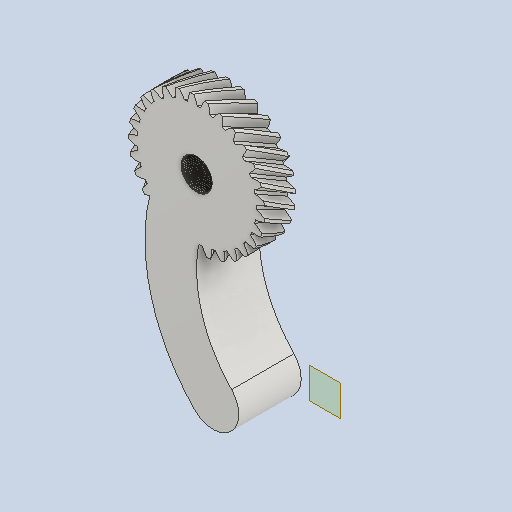
# Autodesk Inventor part: Spur Gear2
Saved by Autodesk Inventor 2024 (Build 280153000, 153)
## iProperties
CustomPartVersion: 1
Created: 2023-09-14
Part Number: Spur Gear2
Material: Steel
Document SubType Name: Modeling
Designer: jebes windows
Categories: <?xml version="1.0" encoding="UTF-16"?> <MemberInstance><Categories><FamilyTemplate><FamilyTemplateParameter ValueType="xs:double" Id="1" ObjectReferenceKey="da_z" ObjectType="kUserParameterObject"/><FamilyTemplateParameter ValueType="xs:double" Id="2" ObjectReferenceKey="da_b" ObjectType="kUserParameterObject"/><FamilyTemplateParameter ValueType="xs:double" Id="3" ObjectReferenceKey="da_beta" ObjectType="kUserParameterObject"/><FamilyTemplateParameter ValueType="xs:double" Id="4" ObjectReferenceKey="da_da" ObjectType="kUserParameterObject"/><FamilyTemplateParameter ValueType="xs:double" Id="5" ObjectReferenceKey="da_aw" ObjectType="kUserParameterObject"/><FamilyTemplateParameter ValueType="xs:string" Id="6" ObjectReferenceKey="EAIAABAAAACIAQAAAAAAAIAAAAAAAAAA" ObjectType="83910656" SubObjectId="SurfaceGeometry"/></FamilyTemplate><ParamToTemplateMap><ParamToTemplate CategoryParameter="//CategoryParameter[@InternalName='046C89C9-8512-4d59-83FE-43B91F4F132A']" TemplateParameter="1"/><ParamToTemplate CategoryParameter="//CategoryParameter[@InternalName='2552DF32-E462-4b46-AEBF-C6C7768E72AC']" TemplateParameter="2"/><ParamToTemplate CategoryParameter="//CategoryParameter[@InternalName='C9EE641D-15FC-4fae-A226-E94C4372FDD7']" TemplateParameter="3"/><ParamToTemplate><ParamToTemplate CategoryParameter="//CategoryParameter[@InternalName='00B6519A-459B-49c7-AD84-2E56D39A5744']" ConstantValue="0.433554"/></ParamToTemplate><ParamToTemplate><ParamToTemplate CategoryParameter="//CategoryParameter[@InternalName='04B31F0E-C7A6-4894-AA32-9629BEFACF47']" ConstantValue="1.000000"/></ParamToTemplate><ParamToTemplate><ParamToTemplate CategoryParameter="//CategoryParameter[@InternalName='43CBEC2E-7847-49e7-A936-2F7889FCB2D9']" ConstantValue="0.250000"/></ParamToTemplate><ParamToTemplate><ParamToTemplate CategoryParameter="//CategoryParameter[@InternalName='B1EFC894-105D-4ebd-86BF-FA20ED196853']" ConstantValue="0.302500"/></ParamToTemplate><ParamToTemplate><ParamToTemplate CategoryParameter="//CategoryParameter[@InternalName='51175063-3D10-4879-93E8-6246FE8B403D']" ConstantValue="2060000000.000000"/></ParamToTemplate><ParamToTemplate><ParamToTemplate CategoryParameter="//CategoryParameter[@InternalName='A3A52E27-4454-46a9-B0BD-C932399B70AF']" ConstantValue="0.300000"/></ParamToTemplate><ParamToTemplate><ParamToTemplate CategoryParameter="//CategoryParameter[@InternalName='91B76062-C214-41d9-B1B9-14D2AB99603D']" ConstantValue="0.060000"/></ParamToTemplate><ParamToTemplate><ParamToTemplate CategoryParameter="//CategoryParameter[@InternalName='374E806E-8B8A-4dda-A9AA-1039D6500AD2']" ConstantValue="16.666667"/></ParamToTemplate><ParamToTemplate><ParamToTemplate CategoryParameter="//CategoryParameter[@InternalName='2D373A89-B862-43d6-8D0B-0CBF12AB9F6C']" ConstantValue="0.436332"/></ParamToTemplate><ParamToTemplate CategoryParameter="//CategoryParameter[@InternalName='37777632-D6A2-4fac-9D53-DB8ACD95C989']" TemplateParameter="4"/><ParamToTemplate CategoryParameter="//CategoryParameter[@InternalName='FD1017F1-B727-4f7e-9707-0F86F1FF9423']" TemplateParameter="5"/><ParamToTemplate><ParamToTemplate CategoryParameter="//CategoryParameter[@InternalName='9E1B4470-B2D3-4ff1-B813-535BB4CDF51A']" ConstantValue="3520000.000000"/></ParamToTemplate><ParamToTemplate><ParamToTemplate CategoryParameter="//CategoryParameter[@InternalName='F8452263-BFF6-458c-9FB1-07C4B99E95CD']" ConstantValue="11400000.000000"/></ParamToTemplate><ParamToTemplate><ParamToTemplate CategoryParameter="//CategoryParameter[@InternalName='3E3BB259-FD49-497f-8171-6EBC954A3479']" ConstantValue="2.000000"/></ParamToTemplate><ParamToTemplate CategoryParameter="//CategoryParameter[@InternalName='27C3BAF2-7550-4e4b-AE2C-0DB134B7D9B7']" TemplateParameter="6"/></ParamToTemplateMap><Category DisplayName="Gear" InternalName="DC85795E-93AB-48d5-8EEE-5A27447B64BD" Mnemonic="Gear"><CategoryParameter DisplayName="z" InternalName="046C89C9-8512-4d59-83FE-43B91F4F132A" Mnemonic="z"/><CategoryParameter DisplayName="b" InternalName="2552DF32-E462-4b46-AEBF-C6C7768E72AC" Mnemonic="b"/><CategoryParameter DisplayName="||b|" InternalName="C9EE641D-15FC-4fae-A226-E94C4372FDD7" Mnemonic="beta"/><CategoryParameter DisplayName="x" InternalName="00B6519A-459B-49c7-AD84-2E56D39A5744" Mnemonic="x"/><CategoryParameter DisplayName="a*" InternalName="04B31F0E-C7A6-4894-AA32-9629BEFACF47" Mnemonic="a"/><CategoryParameter DisplayName="c*" InternalName="43CBEC2E-7847-49e7-A936-2F7889FCB2D9" Mnemonic="c"/><CategoryParameter DisplayName="r|.f|*" InternalName="B1EFC894-105D-4ebd-86BF-FA20ED196853" Mnemonic="rf"/><CategoryParameter DisplayName="E" InternalName="51175063-3D10-4879-93E8-6246FE8B403D" Mnemonic="E"/><CategoryParameter DisplayName="||m|" InternalName="A3A52E27-4454-46a9-B0BD-C932399B70AF" Mnemonic="mi"/><Category DisplayName="SpurGear" InternalName="26C5A22E-A91E-4dfd-A3B3-23CCAFAE1764" Mnemonic="SpurGear"><CategoryParameter DisplayName="m" InternalName="91B76062-C214-41d9-B1B9-14D2AB99603D" Mnemonic="m"/><CategoryParameter DisplayName="P" InternalName="374E806E-8B8A-4dda-A9AA-1039D6500AD2" Mnemonic="PP"/><CategoryParameter DisplayName="||a|" InternalName="2D373A89-B862-43d6-8D0B-0CBF12AB9F6C" Mnemonic="alpha"/><CategoryParameter DisplayName="d|.a|" InternalName="37777632-D6A2-4fac-9D53-DB8ACD95C989" Mnemonic="da"/><CategoryParameter DisplayName="a|.w|" InternalName="FD1017F1-B727-4f7e-9707-0F86F1FF9423" Mnemonic="aw"/><CategoryParameter DisplayName="||s||.Flim|" InternalName="9E1B4470-B2D3-4ff1-B813-535BB4CDF51A" Mnemonic="sFlim"/><CategoryParameter DisplayName="||s||.Hlim|" InternalName="F8452263-BFF6-458c-9FB1-07C4B99E95CD" Mnemonic="sHlim"/><CategoryParameter DisplayName="type" InternalName="3E3BB259-FD49-497f-8171-6EBC954A3479" Mnemonic="type"/><CategoryParameter DisplayName="PitchDiameter" InternalName="27C3BAF2-7550-4e4b-AE2C-0DB134B7D9B7" Mnemonic="IDS_PITCHDIAM"/></Category></Category></Categories></MemberInstance>
Density: 1 g/cm^3
Appearance: Steel
Author: jebes windows
## iProperties of the stored document Spur Gear22_3DPrint.ipt
Created: 2023-09-14
Part Number: Spur Gear22_3DPrint
Material: Generic
Document SubType Name: Modeling
Designer: jebes windows
Density: 1 g/cm^3
Appearance: Default
Author: jebes windows
Autodesk Inventor part; units mm, degrees
ref_plane "YZ Plane" through (0, 0, 0) normal (1, 0, 0) x (0, 1, 0)
ref_plane "XZ Plane" through (0, 0, 0) normal (0, 1, 0) x (-1, 0, 0)
ref_plane "XY Plane" through (0, 0, 0) normal (0, 0, 1) x (1, 0, 0)
sketch "Sketch1" plane through (0, 0, 0) normal (0, 0, 1) x (1, 0, 0)
  circle A0 centre (0, 0) radius 10.9005
  dimension "d0" = 21.801
  constraints: 1 centre point
  measures "d0" diameter of A0
extrude "Extrusion1" add sketch "Sketch1" along normal blind 5
ref_plane "Work Plane2" through (0, 0, 2.5) normal (0, 0, 1) x (1, 0, 0)
sketch "Sketch2" plane through (0, 0, 0) normal (0, 0, -1) x (-1, 0, 0)
  circle A0 centre (0, 0) radius 10.9005 projected
  circle A1 centre (0, 0) radius 10.0459
  dimension "d3" = 20.0918
  constraints: 1 centre point, 1 coincident
  measures "d3" diameter of A1
surface extrude "Pitch Diameter" sketch "Sketch2" against normal through all shown no curves A1
ref_plane "Work Plane8" through (0, 0, 0) normal (0.994138, 0.108119, 0) x (0, 0, 1)
ref_plane "Work Plane9" through (0, 0, 0) normal (1, 0, 0) x (0, 1, 0)
spur gear teeth "Spur Gear" teeth 29 pitch diameter 20.0918 tip diameter 21.801 root diameter 19.1121 face width 5 helix angle 30 hand right start plane through (0, 0, 0) normal (0, 0, -1) x (-1, 0, 0)
sketch "Sketch3" plane through (0, 0, 0) normal (0, 0, -1) x (-1, 0, 0)
  circle A0 centre (0, 0) radius 2.5
  dimension "d49" = 5
  constraints: 1 centre point, 1 coincident
  measures "d49" diameter of A0
extrude "Extrusion2" cut sketch "Sketch3" against normal blind 10
ref_plane "Work Plane11" through (17.5512, -23.0514, 1.9) normal (0, 0, -1) x (0, 1, 0)
sketch "Sketch4" plane through (17.5512, -23.0514, 1.9) normal (0, 0, -1) x (0, 1, 0)
  line L0 (25.1983, -18.5069) -> (25.3277, -18.4572) projected
  arc A0 (25.3277, -18.4572) -> (25.3493, -18.4008) centre (23.0514, -17.5512) ccw projected
  line L1 (25.3493, -18.4008) -> (25.2864, -18.2773) projected
  line L2 (25.2864, -18.2773) -> (25.4099, -18.2143) projected
  arc A1 (25.4099, -18.2143) -> (25.4256, -18.1559) centre (23.0514, -17.5512) ccw projected
  line L3 (25.4256, -18.1559) -> (25.35, -18.0397) projected
  line L4 (25.35, -18.0397) -> (25.4663, -17.9641) projected
  arc A2 (25.4663, -17.9641) -> (25.4758, -17.9045) centre (23.0514, -17.5512) ccw projected
  line L5 (25.4758, -17.9045) -> (25.3885, -17.7967) projected
  line L6 (25.3885, -17.7967) -> (25.4963, -17.7095) projected
  arc A3 (25.4963, -17.7095) -> (25.4994, -17.6491) centre (23.0514, -17.5512) ccw projected
  line L7 (25.4994, -17.6491) -> (25.4014, -17.5511) projected
  line L8 (25.4014, -17.5511) -> (25.4994, -17.453) projected
  arc A4 (25.4994, -17.453) -> (25.4962, -17.3927) centre (23.0514, -17.5512) ccw projected
  line L9 (25.4962, -17.3927) -> (25.3885, -17.3054) projected
  line L10 (25.3885, -17.3054) -> (25.4757, -17.1977) projected
  arc A5 (25.4757, -17.1977) -> (25.4663, -17.138) centre (23.0514, -17.5512) ccw projected
  line L11 (25.4663, -17.138) -> (25.35, -17.0625) projected
  line L12 (25.35, -17.0625) -> (25.4255, -16.9462) projected
  arc A6 (25.4255, -16.9462) -> (25.4099, -16.8878) centre (23.0514, -17.5512) ccw projected
  line L13 (25.4099, -16.8878) -> (25.2863, -16.8249) projected
  line L14 (25.2863, -16.8249) -> (25.3493, -16.7014) projected
  arc A7 (25.3493, -16.7014) -> (25.3276, -16.6449) centre (23.0514, -17.5512) ccw projected
  line L15 (25.3276, -16.6449) -> (25.1982, -16.5953) projected
  line L16 (25.1982, -16.5953) -> (25.2478, -16.4658) projected
  arc A8 (25.2478, -16.4658) -> (25.2204, -16.412) centre (23.0514, -17.5512) ccw projected
  line L17 (25.2204, -16.412) -> (25.0865, -16.3761) projected
  line L18 (25.0865, -16.3761) -> (25.1224, -16.2422) projected
  circle A9 centre (23.0514, -17.5512) radius 2.5 projected
  circle A10 centre (23.0514, -17.5512) radius 0.8 projected
  arc A11 (25.1224, -16.2422) -> (25.0894, -16.1915) centre (23.0514, -17.5512) ccw projected
  line L19 (25.0894, -16.1915) -> (24.9525, -16.1698) projected
  line L20 (24.9525, -16.1698) -> (24.9742, -16.0329) projected
  arc A12 (24.9742, -16.0329) -> (24.9361, -15.9859) centre (23.0514, -17.5512) ccw projected
  line L21 (24.9361, -15.9859) -> (24.7977, -15.9786) projected
  line L22 (24.7977, -15.9786) -> (24.8049, -15.8402) projected
  arc A13 (24.8049, -15.8402) -> (24.7622, -15.7975) centre (23.0514, -17.5512) ccw projected
  circle A14 centre (23.0514, -17.5512) radius 2.5 projected
  circle A15 centre (23.0514, -17.5512) radius 0.8 projected
  line L23 (24.7622, -15.7975) -> (24.6237, -15.8047) projected
  line L24 (24.6237, -15.8047) -> (24.6165, -15.6663) projected
  arc A16 (24.6165, -15.6663) -> (24.5695, -15.6282) centre (23.0514, -17.5512) ccw projected
  line L25 (24.5695, -15.6282) -> (24.4326, -15.6499) projected
  line L26 (24.4326, -15.6499) -> (24.4109, -15.513) projected
  arc A17 (24.4109, -15.513) -> (24.3602, -15.4801) centre (23.0514, -17.5512) ccw projected
  line L27 (24.3602, -15.4801) -> (24.2263, -15.516) projected
  line L28 (24.2263, -15.516) -> (24.1904, -15.382) projected
  arc A18 (24.1904, -15.382) -> (24.1365, -15.3546) centre (23.0514, -17.5512) ccw projected
  line L29 (24.1365, -15.3546) -> (24.0071, -15.4043) projected
  line L30 (24.0071, -15.4043) -> (23.9574, -15.2749) projected
  arc A19 (23.9574, -15.2749) -> (23.901, -15.2532) centre (23.0514, -17.5512) ccw projected
  line L31 (23.901, -15.2532) -> (23.7775, -15.3162) projected
  line L32 (23.7775, -15.3162) -> (23.7145, -15.1926) projected
  arc A20 (23.7145, -15.1926) -> (23.6561, -15.177) centre (23.0514, -17.5512) ccw projected
  line L33 (23.6561, -15.177) -> (23.5399, -15.2525) projected
  line L34 (23.5399, -15.2525) -> (23.4643, -15.1362) projected
  arc A21 (23.4643, -15.1362) -> (23.4046, -15.1268) centre (23.0514, -17.5512) ccw projected
  line L35 (23.4046, -15.1268) -> (23.2969, -15.214) projected
  circle A22 centre (23.0514, -17.5512) radius 2.5 projected
  circle A23 centre (23.0514, -17.5512) radius 0.8 projected
  line L36 (23.2969, -15.214) -> (23.2096, -15.1063) projected
  arc A24 (23.2096, -15.1063) -> (23.1493, -15.1031) centre (23.0514, -17.5512) ccw projected
  line L37 (23.1493, -15.1031) -> (23.0513, -15.2012) projected
  line L38 (23.0513, -15.2012) -> (22.9532, -15.1032) projected
  arc A25 (22.9532, -15.1032) -> (22.8929, -15.1063) centre (23.0514, -17.5512) ccw projected
  line L39 (22.8929, -15.1063) -> (22.8056, -15.2141) projected
  line L40 (22.8056, -15.2141) -> (22.6979, -15.1268) projected
  arc A26 (22.6979, -15.1268) -> (22.6382, -15.1363) centre (23.0514, -17.5512) ccw projected
  line L41 (22.6382, -15.1363) -> (22.5627, -15.2526) projected
  line L42 (22.5627, -15.2526) -> (22.4464, -15.1771) projected
  arc A27 (22.4464, -15.1771) -> (22.388, -15.1927) centre (23.0514, -17.5512) ccw projected
  line L43 (22.388, -15.1927) -> (22.3251, -15.3162) projected
  line L44 (22.3251, -15.3162) -> (22.2015, -15.2533) projected
  arc A28 (22.2015, -15.2533) -> (22.1451, -15.275) centre (23.0514, -17.5512) ccw projected
  line L45 (22.1451, -15.275) -> (22.0954, -15.4044) projected
  circle A29 centre (23.0514, -17.5512) radius 2.5 projected
  circle A30 centre (23.0514, -17.5512) radius 0.8 projected
  line L46 (22.0954, -15.4044) -> (21.966, -15.3547) projected
  arc A31 (21.966, -15.3547) -> (21.9122, -15.3822) centre (23.0514, -17.5512) ccw projected
  line L47 (21.9122, -15.3822) -> (21.8763, -15.5161) projected
  line L48 (21.8763, -15.5161) -> (21.7424, -15.4802) projected
  arc A32 (21.7424, -15.4802) -> (21.6917, -15.5131) centre (23.0514, -17.5512) ccw projected
  line L49 (21.6917, -15.5131) -> (21.67, -15.6501) projected
  line L50 (21.67, -15.6501) -> (21.533, -15.6284) projected
  arc A33 (21.533, -15.6284) -> (21.4861, -15.6664) centre (23.0514, -17.5512) ccw projected
  line L51 (21.4861, -15.6664) -> (21.4788, -15.8049) projected
  line L52 (21.4788, -15.8049) -> (21.3404, -15.7976) projected
  arc A34 (21.3404, -15.7976) -> (21.2976, -15.8404) centre (23.0514, -17.5512) ccw projected
  line L53 (21.2976, -15.8404) -> (21.3049, -15.9788) projected
  line L54 (21.3049, -15.9788) -> (21.1665, -15.9861) projected
  arc A35 (21.1665, -15.9861) -> (21.1284, -16.033) centre (23.0514, -17.5512) ccw projected
  line L55 (21.1284, -16.033) -> (21.1501, -16.17) projected
  line L56 (21.1501, -16.17) -> (21.0132, -16.1917) projected
  arc A36 (21.0132, -16.1917) -> (20.9803, -16.2424) centre (23.0514, -17.5512) ccw projected
  line L57 (20.9803, -16.2424) -> (21.0162, -16.3763) projected
  line L58 (21.0162, -16.3763) -> (20.8822, -16.4122) projected
  circle A37 centre (23.0514, -17.5512) radius 2.5 projected
  circle A38 centre (23.0514, -17.5512) radius 0.8 projected
  arc A39 (20.8822, -16.4122) -> (20.8548, -16.466) centre (23.0514, -17.5512) ccw projected
  line L59 (20.8548, -16.466) -> (20.9045, -16.5955) projected
  line L60 (20.9045, -16.5955) -> (20.7751, -16.6452) projected
  arc A40 (20.7751, -16.6452) -> (20.7534, -16.7016) centre (23.0514, -17.5512) ccw projected
  line L61 (20.7534, -16.7016) -> (20.8164, -16.8251) projected
  line L62 (20.8164, -16.8251) -> (20.6928, -16.8881) projected
  circle A41 centre (23.0514, -17.5512) radius 2.5 projected
  circle A42 centre (23.0514, -17.5512) radius 0.8 projected
  arc A43 (20.6928, -16.8881) -> (20.6772, -16.9464) centre (23.0514, -17.5512) ccw projected
  line L63 (20.6772, -16.9464) -> (20.7527, -17.0627) projected
  line L64 (20.7527, -17.0627) -> (20.6364, -17.1382) projected
  arc A44 (20.6364, -17.1382) -> (20.627, -17.1979) centre (23.0514, -17.5512) ccw projected
  line L65 (20.627, -17.1979) -> (20.7142, -17.3057) projected
  line L66 (20.7142, -17.3057) -> (20.6065, -17.3929) projected
  arc A45 (20.6065, -17.3929) -> (20.6033, -17.4533) centre (23.0514, -17.5512) ccw projected
  line L67 (20.6033, -17.4533) -> (20.7014, -17.5513) projected
  line L68 (20.7014, -17.5513) -> (20.6033, -17.6493) projected
  arc A46 (20.6033, -17.6493) -> (20.6065, -17.7097) centre (23.0514, -17.5512) ccw projected
  line L69 (20.6065, -17.7097) -> (20.7143, -17.7969) projected
  line L70 (20.7143, -17.7969) -> (20.627, -17.9047) projected
  arc A47 (20.627, -17.9047) -> (20.6365, -17.9644) centre (23.0514, -17.5512) ccw projected
  line L71 (20.6365, -17.9644) -> (20.7528, -18.0399) projected
  line L72 (20.7528, -18.0399) -> (20.6772, -18.1562) projected
  arc A48 (20.6772, -18.1562) -> (20.6929, -18.2145) centre (23.0514, -17.5512) ccw projected
  line L73 (20.6929, -18.2145) -> (20.8164, -18.2775) projected
  line L74 (20.8164, -18.2775) -> (20.7535, -18.401) projected
  arc A49 (20.7535, -18.401) -> (20.7752, -18.4574) centre (23.0514, -17.5512) ccw projected
  line L75 (20.7752, -18.4574) -> (20.9046, -18.5071) projected
  line L76 (20.9046, -18.5071) -> (20.8549, -18.6366) projected
  arc A50 (20.8549, -18.6366) -> (20.8823, -18.6904) centre (23.0514, -17.5512) ccw projected
  line L77 (20.8823, -18.6904) -> (21.0163, -18.7263) projected
  line L78 (21.0163, -18.7263) -> (20.9804, -18.8602) projected
  arc A51 (20.9804, -18.8602) -> (21.0133, -18.9109) centre (23.0514, -17.5512) ccw projected
  line L79 (21.0133, -18.9109) -> (21.1503, -18.9326) projected
  line L80 (21.1503, -18.9326) -> (21.1286, -19.0695) projected
  arc A52 (21.1286, -19.0695) -> (21.1666, -19.1165) centre (23.0514, -17.5512) ccw projected
  line L81 (21.1666, -19.1165) -> (21.3051, -19.1237) projected
  line L82 (21.3051, -19.1237) -> (21.2978, -19.2622) projected
  arc A53 (21.2978, -19.2622) -> (21.3405, -19.3049) centre (23.0514, -17.5512) ccw projected
  line L83 (21.3405, -19.3049) -> (21.479, -19.2977) projected
  line L84 (21.479, -19.2977) -> (21.4863, -19.4361) projected
  arc A54 (21.4863, -19.4361) -> (21.5332, -19.4741) centre (23.0514, -17.5512) ccw projected
  line L85 (21.5332, -19.4741) -> (21.6702, -19.4524) projected
  line L86 (21.6702, -19.4524) -> (21.6919, -19.5894) projected
  arc A55 (21.6919, -19.5894) -> (21.7426, -19.6223) centre (23.0514, -17.5512) ccw projected
  line L87 (21.7426, -19.6223) -> (21.8765, -19.5864) projected
  line L88 (21.8765, -19.5864) -> (21.9124, -19.7203) projected
  arc A56 (21.9124, -19.7203) -> (21.9662, -19.7478) centre (23.0514, -17.5512) ccw projected
  line L89 (21.9662, -19.7478) -> (22.0956, -19.6981) projected
  line L90 (22.0956, -19.6981) -> (22.1453, -19.8275) projected
  arc A57 (22.1453, -19.8275) -> (22.2018, -19.8492) centre (23.0514, -17.5512) ccw projected
  line L91 (22.2018, -19.8492) -> (22.3253, -19.7862) projected
  line L92 (22.3253, -19.7862) -> (22.3882, -19.9097) projected
  arc A58 (22.3882, -19.9097) -> (22.4466, -19.9254) centre (23.0514, -17.5512) ccw projected
  line L93 (22.4466, -19.9254) -> (22.5629, -19.8499) projected
  line L94 (22.5629, -19.8499) -> (22.6384, -19.9661) projected
  arc A59 (22.6384, -19.9661) -> (22.6981, -19.9756) centre (23.0514, -17.5512) ccw projected
  line L95 (22.6981, -19.9756) -> (22.8058, -19.8883) projected
  line L96 (22.8058, -19.8883) -> (22.8931, -19.9961) projected
  circle A60 centre (23.0514, -17.5512) radius 2.5 projected
  circle A61 centre (23.0514, -17.5512) radius 0.8 projected
  line L97 (22.9535, -19.9992) -> (23.0515, -19.9012) projected
  arc A62 (22.8931, -19.9961) -> (22.9535, -19.9992) centre (23.0514, -17.5512) ccw projected
  line L98 (23.0515, -19.9012) -> (23.1495, -19.9992) projected
  arc A63 (23.1495, -19.9992) -> (23.2099, -19.9961) centre (23.0514, -17.5512) ccw projected
  line L99 (23.2099, -19.9961) -> (23.2971, -19.8883) projected
  circle A64 centre (23.0514, -17.5512) radius 2.5 projected
  circle A65 centre (23.0514, -17.5512) radius 0.8 projected
  line L100 (23.2971, -19.8883) -> (23.4049, -19.9755) projected
  arc A66 (23.4049, -19.9755) -> (23.4646, -19.9661) centre (23.0514, -17.5512) ccw projected
  line L101 (23.4646, -19.9661) -> (23.5401, -19.8498) projected
  circle A67 centre (23.0514, -17.5512) radius 2.5 projected
  circle A68 centre (23.0514, -17.5512) radius 0.8 projected
  line L102 (23.5401, -19.8498) -> (23.6564, -19.9253) projected
  arc A69 (23.6564, -19.9253) -> (23.7147, -19.9097) centre (23.0514, -17.5512) ccw projected
  line L103 (23.7147, -19.9097) -> (23.7777, -19.7861) projected
  line L104 (23.7777, -19.7861) -> (23.9012, -19.8491) projected
  arc A70 (23.9012, -19.8491) -> (23.9576, -19.8274) centre (23.0514, -17.5512) ccw projected
  line L105 (23.9576, -19.8274) -> (24.0073, -19.698) projected
  circle A71 centre (23.0514, -17.5512) radius 2.5 projected
  circle A72 centre (23.0514, -17.5512) radius 0.8 projected
  line L106 (24.0073, -19.698) -> (24.1368, -19.7477) projected
  arc A73 (24.1368, -19.7477) -> (24.1906, -19.7202) centre (23.0514, -17.5512) ccw projected
  line L107 (24.1906, -19.7202) -> (24.2265, -19.5863) projected
  line L108 (24.2265, -19.5863) -> (24.3604, -19.6222) projected
  arc A74 (24.3604, -19.6222) -> (24.4111, -19.5893) centre (23.0514, -17.5512) ccw projected
  line L109 (24.4111, -19.5893) -> (24.4328, -19.4523) projected
  circle A75 centre (23.0514, -17.5512) radius 2.5 projected
  circle A76 centre (23.0514, -17.5512) radius 0.8 projected
  line L110 (24.4328, -19.4523) -> (24.5697, -19.474) projected
  arc A77 (24.5697, -19.474) -> (24.6167, -19.436) centre (23.0514, -17.5512) ccw projected
  line L111 (24.6167, -19.436) -> (24.6239, -19.2975) projected
  circle A78 centre (23.0514, -17.5512) radius 2.5 projected
  circle A79 centre (23.0514, -17.5512) radius 0.8 projected
  line L112 (24.6239, -19.2975) -> (24.7624, -19.3048) projected
  arc A80 (24.7624, -19.3048) -> (24.8051, -19.262) centre (23.0514, -17.5512) ccw projected
  line L113 (24.8051, -19.262) -> (24.7978, -19.1236) projected
  line L114 (24.7978, -19.1236) -> (24.9363, -19.1163) projected
  arc A81 (24.9363, -19.1163) -> (24.9743, -19.0693) centre (23.0514, -17.5512) ccw projected
  line L115 (24.9743, -19.0693) -> (24.9526, -18.9324) projected
  line L116 (24.9526, -18.9324) -> (25.0896, -18.9107) projected
  arc A82 (25.0896, -18.9107) -> (25.1225, -18.86) centre (23.0514, -17.5512) ccw projected
  circle A83 centre (23.0514, -17.5512) radius 2.5 projected
  circle A84 centre (23.0514, -17.5512) radius 0.8 projected
  line L117 (25.1225, -18.86) -> (25.0866, -18.7261) projected
  line L118 (25.0866, -18.7261) -> (25.2205, -18.6902) projected
  arc A85 (25.2205, -18.6902) -> (25.2479, -18.6363) centre (23.0514, -17.5512) ccw projected
  line L119 (25.2479, -18.6363) -> (25.1983, -18.5069) projected
  point P0 (23.0514, -17.5512)
extrude "Extrusion3" add sketch "Sketch4" along normal blind 2 and the other way blind 3 contours A9
sketch "Sketch5" plane through (0, 0, 0) normal (0, 0, -1) x (-1, 0, 0)
  circle A0 centre (0, 0) radius 2.5 projected
  arc A1 (2.6307, 10.5783) -> (2.0542, 10.7052) centre (0, 0) ccw projected
  arc A2 (0.2952, 10.8965) -> (-0.2952, 10.8965) centre (0, 0) ccw projected
  arc A3 (-2.0542, 10.7052) -> (-2.6307, 10.5783) centre (0, 0) ccw projected
  arc A4 (-4.3074, 10.0134) -> (-4.8432, 9.7655) centre (0, 0) ccw projected
  arc A5 (-6.3593, 8.8533) -> (-6.8293, 8.496) centre (0, 0) ccw projected
  arc A6 (-8.1138, 7.2792) -> (-8.496, 6.8293) centre (0, 0) ccw projected
  arc A7 (-9.4889, 5.3648) -> (-9.7655, 4.8432) centre (0, 0) ccw projected
  arc A8 (-10.4204, 3.1995) -> (-10.5783, 2.6307) centre (0, 0) ccw projected
  arc A9 (-10.8646, 0.8847) -> (-10.8965, 0.2952) centre (0, 0) ccw projected
  arc A10 (-10.8007, -1.4716) -> (-10.7052, -2.0542) centre (0, 0) ccw projected
  arc A11 (-10.2319, -3.759) -> (-10.0134, -4.3074) centre (0, 0) ccw projected
  arc A12 (-9.1846, -5.8707) -> (-8.8533, -6.3593) centre (0, 0) ccw projected
  arc A13 (-7.7078, -7.7078) -> (-7.2792, -8.1138) centre (0, 0) ccw projected
  arc A14 (-5.8707, -9.1846) -> (-5.3648, -9.4889) centre (0, 0) ccw projected
  arc A15 (-3.759, -10.2319) -> (-3.1995, -10.4204) centre (0, 0) ccw projected
  arc A16 (-1.4716, -10.8007) -> (-0.8847, -10.8646) centre (0, 0) ccw projected
  arc A17 (0.8847, -10.8646) -> (1.4716, -10.8007) centre (0, 0) ccw projected
  arc A18 (3.1995, -10.4204) -> (3.759, -10.2319) centre (0, 0) ccw projected
  arc A19 (5.3648, -9.4889) -> (5.8707, -9.1846) centre (0, 0) ccw projected
  arc A20 (7.2792, -8.1138) -> (7.7078, -7.7078) centre (0, 0) ccw projected
  arc A21 (8.8533, -6.3593) -> (9.1846, -5.8707) centre (0, 0) ccw projected
  arc A22 (10.0134, -4.3074) -> (10.2319, -3.759) centre (0, 0) ccw projected
  arc A23 (10.7052, -2.0542) -> (10.8007, -1.4716) centre (0, 0) ccw projected
  arc A24 (10.8965, 0.2952) -> (10.8646, 0.8847) centre (0, 0) ccw projected
  arc A25 (10.5783, 2.6307) -> (10.4204, 3.1995) centre (0, 0) ccw projected
  arc A26 (9.7655, 4.8432) -> (9.4889, 5.3648) centre (0, 0) ccw projected
  arc A27 (8.496, 6.8293) -> (8.1138, 7.2792) centre (0, 0) ccw projected
  arc A28 (6.8293, 8.496) -> (6.3593, 8.8533) centre (0, 0) ccw projected
  arc A29 (4.8432, 9.7655) -> (4.3074, 10.0134) centre (0, 0) ccw projected
  circle A30 centre (-20, -13.2288) radius 20
  line L0 (0, 0) -> (-5, 0)
  line L1 (0, 0) -> (5, 0)
  circle A31 centre (-20, -13.2288) radius 28.2843
  circle A32 centre (-2.6343, -30) radius 4.1421
  point P0 (-5.6138, -27.1225)
  point P1 (0.3452, -32.8775)
  point P2 (2.5, 0)
  point P3 (-2.5, 0)
  dimension "d56" = 40
  dimension "d57" = 5
  dimension "d58" = 5
  dimension "d59" = 20
  dimension "d60" = 56.5685
  dimension "d61" = 30
  constraints: 4 end point, 2 centre point, 2 horizontal, 1 horizontal alignment, 1 tangent, 90 other
  measures "d57" distance of L0.start L0.end
  measures "d58" distance of L0.start L1.end
  measures "d59" horizontal distance of point (0, 0) A31.centre
  measures "d60" diameter of A31
  measures "d61" vertical distance of A32.centre point (0, 0)
extrude "Extrusion4" add sketch "Sketch5" along normal mid plane 10 contours L1 A31 A32 A30 L0 A0 | A32 picked at (5.3496, -15.0279)
equation "\"d0\" = da_da"
equation "\"d1\" = da_b"
equation "\"d3\" = da_d"
equation "\"da_da\" = 21.801031"
equation "\"da_b\" = 5"
equation "\"da_d\" = 20.091789"
body "Solid1"
body "Srf1"
